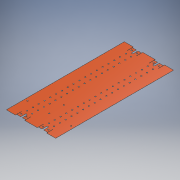
# Autodesk Inventor part: Skin NPS 6
Saved by Autodesk Inventor 2019 (Build 230136000, 136)
## iProperties
Created: 2016-08-10
Part Number: Skin NPS 6
Material: Rubber, Silicone
Document SubType Name: Modeling
Designer: IEUser
Density: 1.25 g/cm^3
Appearance: Rubber - Black
Author: IEUser
Autodesk Inventor part; units mm, degrees
ref_plane "YZ Plane" through (0, 0, 0) normal (1, 0, 0) x (0, 1, 0)
ref_plane "XZ Plane" through (0, 0, 0) normal (0, 1, 0) x (-1, 0, 0)
ref_plane "XY Plane" through (0, 0, 0) normal (0, 0, 1) x (1, 0, 0)
sketch "Skin Scheme" plane through (0, 0, 0) normal (0, 1, 0) x (-1, 0, 0)
  line L0 (647, -212) -> (-647, -212)
  line L1 (-647, -212) -> (-647, 212)
  line L2 (-647, 212) -> (647, 212)
  line L3 (647, 212) -> (647, -212)
  circle A0 centre (475, -116) radius 5
  circle A1 centre (475, -72) radius 5
  circle A2 centre (475, 72) radius 5
  circle A3 centre (475, 116) radius 5
  circle A4 centre (425, -116) radius 5
  circle A5 centre (425, -72) radius 5
  circle A6 centre (425, 72) radius 5
  circle A7 centre (425, 116) radius 5
  circle A8 centre (375, -116) radius 5
  circle A9 centre (375, -72) radius 5
  circle A10 centre (375, 72) radius 5
  circle A11 centre (375, 116) radius 5
  circle A12 centre (325, -116) radius 5
  circle A13 centre (325, -72) radius 5
  circle A14 centre (325, 72) radius 5
  circle A15 centre (325, 116) radius 5
  circle A16 centre (275, -116) radius 5
  circle A17 centre (275, -72) radius 5
  circle A18 centre (275, 72) radius 5
  circle A19 centre (275, 116) radius 5
  circle A20 centre (225, -116) radius 5
  circle A21 centre (225, -72) radius 5
  circle A22 centre (225, 72) radius 5
  circle A23 centre (225, 116) radius 5
  circle A24 centre (175, -116) radius 5
  circle A25 centre (175, -72) radius 5
  circle A26 centre (175, 72) radius 5
  circle A27 centre (175, 116) radius 5
  circle A28 centre (125, -116) radius 5
  circle A29 centre (125, -72) radius 5
  circle A30 centre (125, 72) radius 5
  circle A31 centre (125, 116) radius 5
  circle A32 centre (75, -116) radius 5
  circle A33 centre (75, -72) radius 5
  circle A34 centre (75, 72) radius 5
  circle A35 centre (75, 116) radius 5
  circle A36 centre (25, -116) radius 5
  circle A37 centre (25, -72) radius 5
  circle A38 centre (25, 72) radius 5
  circle A39 centre (25, 116) radius 5
  circle A40 centre (-25, -116) radius 5
  circle A41 centre (-25, -72) radius 5
  circle A42 centre (-25, 72) radius 5
  circle A43 centre (-25, 116) radius 5
  circle A44 centre (-75, -116) radius 5
  circle A45 centre (-75, -72) radius 5
  circle A46 centre (-75, 72) radius 5
  circle A47 centre (-75, 116) radius 5
  circle A48 centre (-125, -116) radius 5
  circle A49 centre (-125, -72) radius 5
  circle A50 centre (-125, 72) radius 5
  circle A51 centre (-125, 116) radius 5
  circle A52 centre (-175, -116) radius 5
  circle A53 centre (-175, -72) radius 5
  circle A54 centre (-175, 72) radius 5
  circle A55 centre (-175, 116) radius 5
  circle A56 centre (-225, -116) radius 5
  circle A57 centre (-225, -72) radius 5
  circle A58 centre (-225, 72) radius 5
  circle A59 centre (-225, 116) radius 5
  circle A60 centre (-275, -116) radius 5
  circle A61 centre (-275, -72) radius 5
  circle A62 centre (-275, 72) radius 5
  circle A63 centre (-275, 116) radius 5
  circle A64 centre (-325, -116) radius 5
  circle A65 centre (-325, -72) radius 5
  circle A66 centre (-325, 72) radius 5
  circle A67 centre (-325, 116) radius 5
  circle A68 centre (-375, -116) radius 5
  circle A69 centre (-375, -72) radius 5
  circle A70 centre (-375, 72) radius 5
  circle A71 centre (-375, 116) radius 5
  circle A72 centre (-425, -116) radius 5
  circle A73 centre (-425, -72) radius 5
  circle A74 centre (-425, 72) radius 5
  circle A75 centre (-425, 116) radius 5
  circle A76 centre (-475, -116) radius 5
  circle A77 centre (-475, -72) radius 5
  circle A78 centre (-475, 72) radius 5
  circle A79 centre (-475, 116) radius 5
  circle A80 centre (350, 0) radius 5
  circle A81 centre (350, -188) radius 5
  circle A82 centre (350, 188) radius 5
  circle A83 centre (225, 0) radius 5
  point P0 (0, 0)
  dimension "d0" = 1294
  dimension "d1" = 647
  dimension "d2" = 424
  dimension "d3" = 212
  dimension "d4" = 10
  dimension "d5" = 172
  dimension "d6" = 96
  dimension "d9" = 44
  dimension "d16" = 188
  dimension "d19" = 50
  dimension "d61" = 25
  dimension "d62" = 72
  dimension "d63" = 72
  dimension "d64" = 25
  dimension "d65" = 72
  dimension "d66" = 25
  dimension "d67" = 10
  dimension "d68" = 10
  dimension "d69" = 10
  dimension "d70" = 250
  dimension "d71" = 0
  dimension "d72" = 10
  constraints: 84 centre point, 8 end point, 2 horizontal, 2 parallel, 2 vertical, 1 perpendicular, 158 other
  measures "d0" distance of L0.start L0.end
  measures "d1" distance from line of point (0, 0) L3
  measures "d2" distance of L2.end L0.start
  measures "d3" distance from line of point (0, 0) L0
  measures "d4" diameter of A0
  measures "d5" distance from line of L3 A0.centre
  measures "d6" distance from line of L0 A0.centre
  measures "d9" distance of A0.centre A1.centre
  measures "d16" distance of A0.centre A2.centre
  measures "d19" distance of A0.centre A4.centre
  measures "d61" horizontal distance of A9.centre A80.centre
  measures "d62" vertical distance of A9.centre A80.centre
  measures "d63" vertical distance of A8.centre A81.centre
  measures "d64" horizontal distance of A81.centre A8.centre
  measures "d65" vertical distance of A11.centre A82.centre
  measures "d66" horizontal distance of A11.centre A82.centre
  measures "d67" diameter of A82
  measures "d68" diameter of A80
  measures "d69" diameter of A81
  measures "d70" horizontal distance of A83.centre A1.centre
  measures "d71" vertical distance of point (0, 0) A83.centre
  measures "d72" diameter of A83
extrude "Skin Body" add sketch "Skin Scheme" along normal blind 1
sketch "Feature Cut Outline" plane through (0, 1, 0) normal (0, 1, 0) x (1, 0, 0)
  circle A0 centre (-475, 116) radius 5 projected
  circle A1 centre (-475, 72) radius 5 projected
  line L0 (-657, 134) -> (-497, 134)
  line L1 (-497, 134) -> (-497, 99)
  line L2 (-497, 99) -> (-457, 99)
  line L3 (-457, 99) -> (-452, 94)
  line L4 (-452, 94) -> (-457, 84)
  line L5 (-457, 84) -> (-497, 84)
  line L6 (-497, 84) -> (-497, 54)
  line L7 (-497, 54) -> (-657, 54)
  line L8 (-657, 54) -> (-657, 134)
  line L9 (-647, 212) -> (-647, -212) projected
  point P0 (0, 0)
  dimension "d33" = 18
  dimension "d34" = 22
  dimension "d35" = 18
  dimension "d36" = 5
  dimension "d37" = 10
  dimension "d38" = 5
  dimension "d39" = 5
  dimension "d40" = 10
  dimension "d41" = 45
  dimension "d42" = 22
  constraints: 18 end point, 3 perpendicular, 2 parallel, 1 collinear, 1 horizontal
  measures "d33" distance from line of A0.centre L0
  measures "d34" distance from line of L1 A0.centre
  measures "d35" distance from line of A1.centre L7
  measures "d36" distance from line of L3.end L2
  measures "d37" distance from line of L3.end L5
  measures "d38" horizontal distance of L4.end L3.end
  measures "d39" horizontal distance of L2.end L3.end
  measures "d40" distance between parallel lines of L9 L8
  measures "d41" distance from line of L6 L3.end
  measures "d42" vertical distance of A1.centre L3.end
extrude "Feature Cut" cut sketch "Feature Cut Outline" along normal through all both and the other way through all contours L0 L9 L7 L8 | L0 L1 L2 L3 L4 L5 L6 L7 L9
mirror "Feature Cut Side Mirror" about plane through (0, 0, 0) normal (0, 0, 1) of "Feature Cut"
mirror "Feature Cut Mirror" about plane through (0, 0, 0) normal (1, 0, 0) of "Feature Cut", "Feature Cut Side Mirror"
sketch "End Cut Outline" plane through (0, 1, 0) normal (0, 1, 0) x (1, 0, 0)
  line L0 (-507, 222) -> (-657, 222)
  line L1 (-657, 222) -> (-657, -222)
  line L2 (-657, -222) -> (-507, -222)
  line L3 (-507, -222) -> (-507, 222)
  line L4 (-647, 212) -> (-647, 134) projected
  line L5 (647, 212) -> (-647, 212) projected
  line L6 (-647, -212) -> (647, -212) projected
  point P0 (0, 0)
  dimension "d45" = 10
  dimension "d46" = 10
  dimension "d47" = 10
  dimension "d48" = 140
  constraints: 8 end point, 2 parallel, 1 horizontal, 1 perpendicular
  measures "d45" distance between parallel lines of L4 L1
  measures "d46" distance between parallel lines of L5 L0
  measures "d47" distance between parallel lines of L2 L6
  measures "d48" distance between parallel lines of L4 L3
extrude "End Cut" cut sketch "End Cut Outline" along normal through all both and the other way through all
mirror "End Cut Mirror" about plane through (0, 0, 0) normal (1, 0, 0) of "End Cut"
sketch "Slot Cut Outline" plane through (0, 1, 0) normal (0, 1, 0) x (1, 0, 0)
  line L0 (-455, 55) -> (-507, 55)
  line L1 (-507, 55) -> (-507, 54)
  line L2 (-507, 54) -> (-455, 54)
  line L3 (-455, 54) -> (-455, 55)
  line L4 (-497, 54) -> (-507, 54) projected
  line L5 (-507, 54) -> (-507, -54) projected
  line L6 (-497, 84) -> (-497, 54) projected
  line L7 (-507, 134) -> (-455, 134)
  line L8 (-455, 134) -> (-455, 133)
  line L9 (-455, 133) -> (-507, 133)
  line L10 (-507, 133) -> (-507, 134)
  line L11 (-507, 134) -> (-497, 134) projected
  line L12 (-497, 134) -> (-497, 99) projected
  line L13 (-507, 212) -> (-507, 134) projected
  point P0 (0, 0)
  dimension "d51" = 0
  dimension "d52" = 1
  dimension "d53" = 0
  dimension "d54" = 42
  dimension "d55" = 0
  dimension "d56" = 1
  dimension "d57" = 42
  dimension "d58" = 0
  constraints: 16 end point, 4 parallel, 2 horizontal, 2 perpendicular
  measures "d51" distance between parallel lines of L4 L2
  measures "d52" distance of L2.end L0.start
  measures "d53" distance between parallel lines of L5 L1
  measures "d54" distance between parallel lines of L6 L3
  measures "d55" distance between parallel lines of L11 L7
  measures "d56" distance of L7.end L8.end
  measures "d57" distance between parallel lines of L12 L8
  measures "d58" distance between parallel lines of L13 L10
extrude "Slot Cut" cut sketch "Slot Cut Outline" along normal through all both and the other way through all
mirror "Slot Cut Side Mirror" about plane through (0, 0, 0) normal (0, 0, 1) of "Slot Cut"
mirror "Slot Cut Mirror" about plane through (0, 0, 0) normal (1, 0, 0) of "Slot Cut", "Slot Cut Side Mirror"
equation "\"d1\" = 0.5 * d0"
equation "\"d3\" = 0.5 * d2"
equation "\"d61\" = 0.5 * d19"
equation "\"d62\" = -0.5 * d9 + 0.5 * d16"
equation "\"d63\" = d62"
equation "\"d64\" = d61"
equation "\"d65\" = d62"
equation "\"d66\" = d61"
equation "\"d67\" = d4"
equation "\"d68\" = d4"
equation "\"d69\" = d4"
equation "\"d70\" = 5 * d19"
equation "\"d56\" = d52"
equation "\"d57\" = d54"
body "Solid1"
